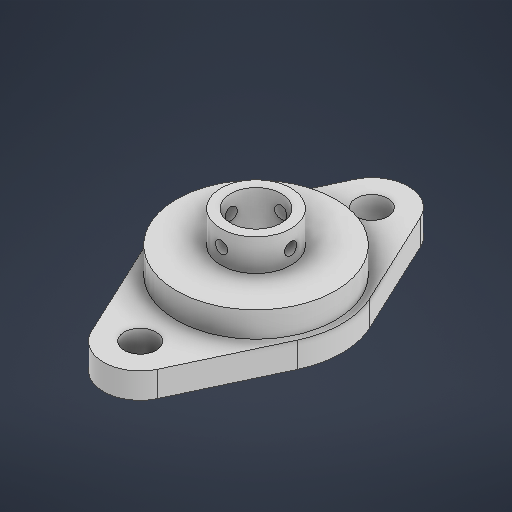
# Autodesk Inventor part: chumacera
Saved by Autodesk Inventor 2025.3 (Build 293356000, 356)
## iProperties
Created: 2025-10-21
Part Number: chumacera
Material: Genérico
Document SubType Name: Modeling
Designer: Jonathan Galarza
Density: 1 g/cm^3
Appearance: Valor por defecto
Author: Jonathan Galarza
Autodesk Inventor part; units mm, degrees
ref_plane "YZ Plane" through (0, 0, 0) normal (1, 0, 0) x (0, 1, 0)
ref_plane "XZ Plane" through (0, 0, 0) normal (0, 1, 0) x (-1, 0, 0)
ref_plane "XY Plane" through (0, 0, 0) normal (0, 0, 1) x (1, 0, 0)
sketch "Boceto1" plane through (0, 0, 0) normal (0, 1, 0) x (-1, 0, 0)
  line L0 (0, 18.25) -> (0, -18.25) construction
  circle A0 centre (0, 18.25) radius 2.5
  circle A1 centre (0, -18.25) radius 2.5
  line L1 (0, 24) -> (0, -24) construction
  arc A2 (5.2058, 20.6918) -> (-5.2058, 20.6918) centre (0, 18.25) ccw
  arc A3 (-5.2058, -20.6918) -> (5.2058, -20.6918) centre (0, -18.25) ccw
  line L2 (12.2223, -5.7329) -> (5.2058, -20.6918)
  line L3 (5.2058, 20.6918) -> (12.2223, 5.7329)
  line L4 (-5.2058, 20.6918) -> (-12.2223, 5.7329)
  line L5 (-12.2223, -5.7329) -> (-5.2058, -20.6918)
  arc A4 (-12.2223, 5.7329) -> (-12.2223, -5.7329) centre (0, 0) ccw
  arc A5 (12.2223, -5.7329) -> (12.2223, 5.7329) centre (0, 0) ccw
  circle A6 centre (0, 0) radius 12.5
  circle A7 centre (0, 0) radius 4
  dimension "d1" = 36.5
  dimension "d2" = 5
  dimension "d3" = 5
  dimension "d4" = 48
  dimension "d5" = 25
  dimension "d6" = 8
  constraints: 12 end point, 10 point on circle, 8 centre point, 8 coincident, 8 tangent, 2 midpoint, 2 vertical
  measures "d1" distance of L0.start L0.end
  measures "d2" diameter of A0
  measures "d3" diameter of A1
  measures "d4" distance of L1.start L1.end
  measures "d5" diameter of A6
  measures "d6" diameter of A7
extrude "Extrusión1" add sketch "Boceto1" against normal blind 4 contours L3 A5 L2 A3 L5 A4 L4 A2 | A6
extrude "Extrusión2" add sketch "Boceto1" along normal blind 4 contours A6
sketch "Boceto2" plane through (0, 4, 0) normal (0, 1, 0) x (1, 0, 0)
  circle A0 centre (0, 0) radius 12.5 projected
  circle A1 centre (0, 0) radius 5.5
  circle A2 centre (0, 0) radius 4 projected
  dimension "d11" = 11
  constraints: 1 centre point, 1 coincident
  measures "d11" diameter of A1
extrude "Extrusión3" add sketch "Boceto2" along normal blind 5 contours A1
sketch "Boceto3" plane through (0, 0, 0) normal (1, 0, 0) x (0, 1, 0)
  circle A0 centre (6.2564, 0) radius 0.95
  point P0 (0, 0)
  dimension "d14" = 1.9
  constraints: 1 centre point
  measures "d14" diameter of A0
extrude "Extrusión4" cut sketch "Boceto3" along normal mid plane 20
sketch "Boceto4" plane through (0, 0, 0) normal (0, 0, 1) x (1, 0, 0)
  circle A0 centre (0, 6.4551) radius 0.95
  point P0 (0, 0)
  dimension "d17" = 1.9
  constraints: 1 centre point
  measures "d17" diameter of A0
extrude "Extrusión5" cut sketch "Boceto4" along normal mid plane 20
sketch "Boceto5" plane through (0, -4, 0) normal (0, -1, 0) x (1, 0, 0)
  circle A0 centre (0, 0) radius 11.15
  circle A1 centre (0, 0) radius 4 projected
  dimension "d20" = 22.3
  constraints: 1 centre point, 1 coincident
  measures "d20" diameter of A0
extrude "Extrusión6" cut sketch "Boceto5" against normal blind 7.1
